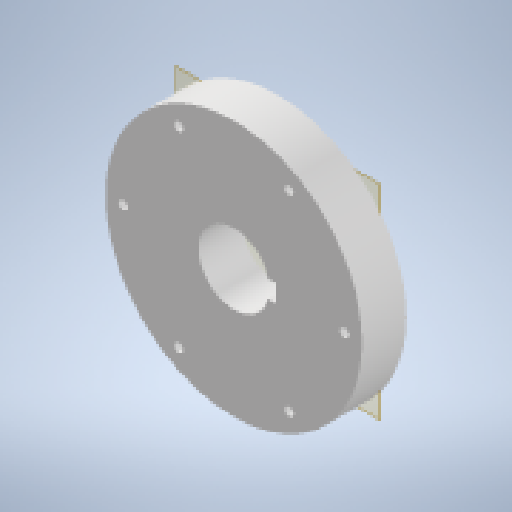
# Autodesk Inventor part: Część6
Saved by Autodesk Inventor 2024 (Build 280153000, 153)
## iProperties
Created: 2023-11-21
Part Number: Część6
Material: Ogólny
Document SubType Name: Modeling
Designer: Wojciech
Density: 1 g/cm^3
Appearance: Domyślna
Author: Wojciech
Autodesk Inventor part; units mm, degrees
ref_plane "YZ Plane" through (0, 0, 0) normal (1, 0, 0) x (0, 1, 0)
ref_plane "XZ Plane" through (0, 0, 0) normal (0, 1, 0) x (-1, 0, 0)
ref_plane "XY Plane" through (0, 0, 0) normal (0, 0, 1) x (1, 0, 0)
ref_plane "Płaszczyzna konstrukcyjna1" through (0, 0, 0) normal (0, 0, 1) x (1, 0, 0)
sketch "Szkic1" plane through (0, 0, 0) normal (0, 0, 1) x (1, 0, 0)
  circle A0 centre (0, 0) radius 72.5 projected
  circle A1 centre (0, 0) radius 35.3971 projected
  arc A2 (19.3649, 5) -> (19.3649, -5) centre (0, 0) ccw projected
  line L0 (24, 5) -> (24, -5) projected
  line L1 (24, -5) -> (19.3649, -5) projected
  line L2 (19.3649, 5) -> (24, 5) projected
extrude "Wyciągnięcie proste1" add sketch "Szkic1" along normal blind 25 contours A0 | A1
sketch "Szkic2" plane through (0, 0, 25) normal (0, 0, 1) x (1, 0, 0)
  circle A0 centre (62.5, 0) radius 2.4585 projected
  point P0 (0, 0)
hole "Otwór1" at (62.5, 0, 25) direction (0, 0, -1) diameter 5 end through all
pattern_circular "Szyk kołowy1" count 6 over 360 about axis through (0, 0, -10) along (0, 0, 1) of "Otwór1"
